belt pully 6mm v2 (Autodesk Fusion 360 design; units mm, degrees)
Autodesk Fusion 360 part; units mm, degrees
sketch "Sketch1" plane through (0, 0, 0) normal (0, 0, 1) x (1, 0, 0)
  circle A0 centre (0, 0) radius 6
  circle A1 centre (0, 0) radius 8.5
  circle A2 centre (0, 0) radius 2.5
  dimension "d1" = 12
  dimension "d2" = 17
  dimension "d3" = 5
  constraint coincident A0.centre A1.centre
  constraint concentric A1 A2
  measures "d1" diameter of A0
  measures "d2" diameter of A1
  measures "d3" diameter of A2
extrude "Extrude1" add sketch "Sketch1" along normal blind 6.5 contours A0
extrude "Extrude2" add sketch "Sketch1" against normal blind 1 contours A0 | A1
sketch "Sketch2" plane through (0, 0, 6.5) normal (0, 0, 1) x (-1, 0, 0)
  circle A0 centre (0, 0) radius 2.5
  circle A1 centre (0, 0) radius 6
  circle A2 centre (0, 0) radius 8.5
  dimension "d8" = 17
  constraint concentric A0 A2
  measures "d8" diameter of A2
extrude "Extrude3" add sketch "Sketch2" along normal blind 1 contours A1 | A2
